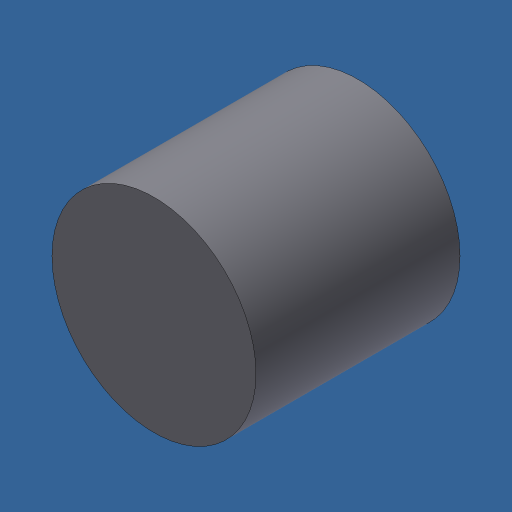
# Autodesk Inventor part: Cylinder, Center Constrained
Saved by Autodesk Inventor 2024.3 (Build 283343000, 343)
## iProperties
Category: _
Manager: _
Created: 2023-11-08
Part Number: Cylinder, Center Constrained
Checked By: 00
Engr Approved By: _
User Status: Work In Process
Material: Steel, MS
Description: CYLINDER, CENTER CONSTRAINED
Document SubType Name: Modeling
Mfg Approved By: Stephen.Oerton
Designer: -
Manufacturer: Standard
Standards Organization: Custom
Mass: 101.161 g
Surface Area: 30.4024 cm^2
Volume: 12.8704 cm^3
Density: 7.86 g/cm^3
Appearance: Metal-Steel
CN_MASS: 0.1
Length: 1.00 in
Diameter: 1.000 in
MaterialSize: =<Diameter> X <Length> Lg
CN_SERVICEABLE: _
CL_runCount: 0
FIRST_DESCRIPTION: _
SECOND_DESCRIPTION: _
THIRD_DESCRIPTION: _
ModelCat: Uncategorized
ILogicPurgeVersion: 2.2.20.20
OnSaveVersion: 2.2.20.20
Subject: _
Author: -
Keywords: -
Revision Number: A
Autodesk Inventor part; units mm, degrees
ref_plane "YZ Plane" through (0, 0, 0) normal (1, 0, 0) x (0, 1, 0)
ref_plane "XZ Plane" through (0, 0, 0) normal (0, 1, 0) x (-1, 0, 0)
ref_plane "XY Plane" through (0, 0, 0) normal (0, 0, 1) x (1, 0, 0)
sketch "Sketch1" plane through (0, 0, 0) normal (0, 0, 1) x (1, 0, 0)
  circle A0 centre (0, 0) radius 12.7
  constraints: 1 centre point, 1 coincident, 1 other
extrude "Extrusion1" add sketch "Sketch1" along normal blind 25.4
